Autodesk Inventor part; units mm, degrees
(part 3 of 3)
sketch "Boceto45" plane through (0, 0, 2) normal (0, 0, 1) x (1, 0, 0)
  line L0 (-14.5048, -25.2952) -> (14.5048, -25.2952) construction
  line L1 (14.5048, -25.2952) -> (14.5048, -27.5438) construction
  line L2 (14.5048, -27.5438) -> (-14.5048, -27.5438) construction
  line L3 (-14.5048, -27.5438) -> (-14.5048, -25.2952) construction
  line L4 (-34, -35) -> (34, -35) projected
  spline S0 degree 2 poles (-12.9457, -26.7231) (-12.9457, -26.8722) (-13.0591, -27.1007) (-13.1531, -27.1753) knots 0 0 0 1 2 2 2
  spline S1 degree 2 poles (-13.1531, -27.1753) (-13.2666, -27.2628) (-13.5243, -27.3374) (-13.7285, -27.3374) knots 0 0 0 1 2 2 2
  line L5 (-13.7285, -27.3374) -> (-14.3022, -27.3374)
  line L6 (-14.3022, -27.3374) -> (-14.3022, -25.3374)
  line L7 (-14.3022, -25.3374) -> (-13.7722, -25.3374)
  spline S2 degree 2 poles (-13.7722, -25.3374) (-13.5583, -25.3374) (-13.3444, -25.3649) (-13.2471, -25.4184) knots 0 0 0 1 2 2 2
  spline S3 degree 2 poles (-13.2471, -25.4184) (-13.1385, -25.4751) (-13.0397, -25.6615) (-13.0397, -25.7879) knots 0 0 0 1 2 2 2
  spline S4 degree 2 poles (-13.0397, -25.7879) (-13.0397, -25.9289) (-13.1888, -26.1526) (-13.32, -26.2158) knots 0 0 0 1 2 2 2
  line L8 (-13.32, -26.2158) -> (-13.32, -26.2255)
  spline S5 degree 2 poles (-13.32, -26.2255) (-13.1418, -26.2741) (-12.9457, -26.5318) (-12.9457, -26.7231) knots 0 0 0 1 2 2 2
  spline S6 degree 2 poles (-13.2228, -26.7344) (-13.2228, -26.621) (-13.2876, -26.4751) (-13.3849, -26.4233) knots 0 0 0 1 2 2 2
  spline S7 degree 2 poles (-13.3849, -26.4233) (-13.4481, -26.3908) (-13.5972, -26.3714) (-13.735, -26.3714) knots 0 0 0 1 2 2 2
  line L9 (-13.735, -26.3714) -> (-14.0364, -26.3714)
  line L10 (-14.0364, -26.3714) -> (-14.0364, -27.1104)
  line L11 (-14.0364, -27.1104) -> (-13.8209, -27.1104)
  spline S8 degree 2 poles (-13.8209, -27.1104) (-13.6458, -27.1104) (-13.4448, -27.078) (-13.367, -27.0262) knots 0 0 0 1 2 2 2
  spline S9 degree 2 poles (-13.367, -27.0262) (-13.2925, -26.9727) (-13.2228, -26.8398) (-13.2228, -26.7344) knots 0 0 0 1 2 2 2
  spline S10 degree 2 poles (-13.3168, -25.8252) (-13.3168, -25.7539) (-13.3654, -25.6469) (-13.4189, -25.6161) knots 0 0 0 1 2 2 2
  spline S11 degree 2 poles (-13.4189, -25.6161) (-13.4837, -25.5805) (-13.6409, -25.5643) (-13.782, -25.5643) knots 0 0 0 1 2 2 2
  line L12 (-13.782, -25.5643) -> (-14.0364, -25.5643)
  line L13 (-14.0364, -25.5643) -> (-14.0364, -26.1493)
  line L14 (-14.0364, -26.1493) -> (-13.735, -26.1493)
  spline S12 degree 2 poles (-13.735, -26.1493) (-13.6102, -26.1493) (-13.4918, -26.1234) (-13.4286, -26.0829) knots 0 0 0 1 2 2 2
  spline S13 degree 2 poles (-13.4286, -26.0829) (-13.367, -26.044) (-13.3168, -25.9192) (-13.3168, -25.8252) knots 0 0 0 1 2 2 2
  spline S14 degree 2 poles (-11.9829, -27.3795) (-12.1596, -27.3795) (-12.4221, -27.2871) (-12.5145, -27.1947) knots 0 0 0 1 2 2 2
  spline S15 degree 2 poles (-12.5145, -27.1947) (-12.6199, -27.091) (-12.7058, -26.7993) (-12.7058, -26.5853) knots 0 0 0 1 2 2 2
  line L15 (-12.7058, -26.5853) -> (-12.7058, -25.3374)
  line L16 (-12.7058, -25.3374) -> (-12.44, -25.3374)
  line L17 (-12.44, -25.3374) -> (-12.44, -26.5853)
  spline S16 degree 2 poles (-12.44, -26.5853) (-12.44, -26.7247) (-12.4043, -26.9127) (-12.3541, -26.9889) knots 0 0 0 1 2 2 2
  spline S17 degree 2 poles (-12.3541, -26.9889) (-12.3006, -27.0699) (-12.1158, -27.1526) (-11.9829, -27.1526) knots 0 0 0 1 2 2 2
  spline S18 degree 2 poles (-11.9829, -27.1526) (-11.8581, -27.1526) (-11.6636, -27.0699) (-11.6102, -26.9889) knots 0 0 0 1 2 2 2
  spline S19 degree 2 poles (-11.6102, -26.9889) (-11.5599, -26.9127) (-11.5243, -26.7263) (-11.5243, -26.5918) knots 0 0 0 1 2 2 2
  line L18 (-11.5243, -26.5918) -> (-11.5243, -25.3374)
  line L19 (-11.5243, -25.3374) -> (-11.2585, -25.3374)
  line L20 (-11.2585, -25.3374) -> (-11.2585, -26.5853)
  spline S20 degree 2 poles (-11.2585, -26.5853) (-11.2585, -26.7944) (-11.3427, -27.0926) (-11.4497, -27.1947) knots 0 0 0 1 2 2 2
  spline S21 degree 2 poles (-11.4497, -27.1947) (-11.5453, -27.2887) (-11.7982, -27.3795) (-11.9829, -27.3795) knots 0 0 0 1 2 2 2
  line L21 (-9.3298, -27.3374) -> (-9.675, -27.3374)
  line L22 (-9.675, -27.3374) -> (-10.3071, -26.5416)
  line L23 (-10.3071, -26.5416) -> (-10.6118, -26.5416)
  line L24 (-10.6118, -26.5416) -> (-10.6118, -27.3374)
  line L25 (-10.6118, -27.3374) -> (-10.8776, -27.3374)
  line L26 (-10.8776, -27.3374) -> (-10.8776, -25.3374)
  line L27 (-10.8776, -25.3374) -> (-10.3622, -25.3374)
  spline S22 degree 2 poles (-10.3622, -25.3374) (-10.1904, -25.3374) (-9.9586, -25.3746) (-9.8533, -25.4427) knots 0 0 0 1 2 2 2
  spline S23 degree 2 poles (-9.8533, -25.4427) (-9.7479, -25.5108) (-9.6264, -25.7231) (-9.6264, -25.8803) knots 0 0 0 1 2 2 2
  spline S24 degree 2 poles (-9.6264, -25.8803) (-9.6264, -26.0991) (-9.85, -26.3957) (-10.0413, -26.467) knots 0 0 0 1 2 2 2
  line L28 (-10.0413, -26.467) -> (-9.3298, -27.3374)
  spline S25 degree 2 poles (-9.9035, -25.9014) (-9.9035, -25.8139) (-9.9651, -25.6793) (-10.0299, -25.6356) knots 0 0 0 1 2 2 2
  spline S26 degree 2 poles (-10.0299, -25.6356) (-10.0867, -25.5983) (-10.2374, -25.5675) (-10.3476, -25.5675) knots 0 0 0 1 2 2 2
  line L29 (-10.3476, -25.5675) -> (-10.6118, -25.5675)
  line L30 (-10.6118, -25.5675) -> (-10.6118, -26.3195)
  line L31 (-10.6118, -26.3195) -> (-10.3784, -26.3195)
  spline S27 degree 2 poles (-10.3784, -26.3195) (-10.2633, -26.3195) (-10.0802, -26.279) (-10.017, -26.2158) knots 0 0 0 1 2 2 2
  spline S28 degree 2 poles (-10.017, -26.2158) (-9.9586, -26.1607) (-9.9035, -26.0051) (-9.9035, -25.9014) knots 0 0 0 1 2 2 2
  line L32 (-7.7398, -27.3374) -> (-8.038, -27.3374)
  line L33 (-8.038, -27.3374) -> (-8.923, -25.6129)
  line L34 (-8.923, -25.6129) -> (-8.923, -27.3374)
  line L35 (-8.923, -27.3374) -> (-9.1709, -27.3374)
  line L36 (-9.1709, -27.3374) -> (-9.1709, -25.3374)
  line L37 (-9.1709, -25.3374) -> (-8.7933, -25.3374)
  line L38 (-8.7933, -25.3374) -> (-7.9878, -26.9208)
  line L39 (-7.9878, -26.9208) -> (-7.9878, -25.3374)
  line L40 (-7.9878, -25.3374) -> (-7.7398, -25.3374)
  line L41 (-7.7398, -25.3374) -> (-7.7398, -27.3374)
  line L42 (-6.6588, -26.5837) -> (-7.4157, -26.5837)
  line L43 (-7.4157, -26.5837) -> (-7.4157, -26.3406)
  line L44 (-7.4157, -26.3406) -> (-6.6588, -26.3406)
  line L45 (-6.6588, -26.3406) -> (-6.6588, -26.5837)
  line L46 (-5.6393, -27.3374) -> (-6.414, -27.3374)
  line L47 (-6.414, -27.3374) -> (-6.414, -27.1331)
  line L48 (-6.414, -27.1331) -> (-6.1596, -27.1331)
  line L49 (-6.1596, -27.1331) -> (-6.1596, -25.5416)
  line L50 (-6.1596, -25.5416) -> (-6.414, -25.5416)
  line L51 (-6.414, -25.5416) -> (-6.414, -25.3374)
  line L52 (-6.414, -25.3374) -> (-5.6393, -25.3374)
  line L53 (-5.6393, -25.3374) -> (-5.6393, -25.5416)
  line L54 (-5.6393, -25.5416) -> (-5.8938, -25.5416)
  line L55 (-5.8938, -25.5416) -> (-5.8938, -27.1331)
  line L56 (-5.8938, -27.1331) -> (-5.6393, -27.1331)
  line L57 (-5.6393, -27.1331) -> (-5.6393, -27.3374)
  line L58 (-3.8792, -27.3374) -> (-4.1774, -27.3374)
  line L59 (-4.1774, -27.3374) -> (-5.0623, -25.6129)
  line L60 (-5.0623, -25.6129) -> (-5.0623, -27.3374)
  line L61 (-5.0623, -27.3374) -> (-5.3103, -27.3374)
  line L62 (-5.3103, -27.3374) -> (-5.3103, -25.3374)
  line L63 (-5.3103, -25.3374) -> (-4.9327, -25.3374)
  line L64 (-4.9327, -25.3374) -> (-4.1272, -26.9208)
  line L65 (-4.1272, -26.9208) -> (-4.1272, -25.3374)
  line L66 (-4.1272, -25.3374) -> (-3.8792, -25.3374)
  line L67 (-3.8792, -25.3374) -> (-3.8792, -27.3374)
  line L68 (-2.1482, -27.3374) -> (-2.1482, -25.574)
  line L69 (-2.1482, -25.574) -> (-2.8192, -25.574)
  line L70 (-2.8192, -25.574) -> (-2.8192, -25.3374)
  line L71 (-2.8192, -25.3374) -> (-1.2115, -25.3374)
  line L72 (-1.2115, -25.3374) -> (-1.2115, -25.574)
  line L73 (-1.2115, -25.574) -> (-1.8824, -25.574)
  line L74 (-1.8824, -25.574) -> (-1.8824, -27.3374)
  line L75 (-1.8824, -27.3374) -> (-2.1482, -27.3374)
  line L76 (-1.0089, -27.3374) -> (-1.0089, -25.3374)
  line L77 (-1.0089, -25.3374) -> (0.2424, -25.3374)
  line L78 (0.2424, -25.3374) -> (0.2424, -25.574)
  line L79 (0.2424, -25.574) -> (-0.7431, -25.574)
  line L80 (-0.7431, -25.574) -> (-0.7431, -26.1218)
  line L81 (-0.7431, -26.1218) -> (0.1759, -26.1218)
  line L82 (0.1759, -26.1218) -> (0.1759, -26.3584)
  line L83 (0.1759, -26.3584) -> (-0.7431, -26.3584)
  line L84 (-0.7431, -26.3584) -> (-0.7431, -27.1007)
  line L85 (-0.7431, -27.1007) -> (0.2424, -27.1007)
  line L86 (0.2424, -27.1007) -> (0.2424, -27.3374)
  line L87 (0.2424, -27.3374) -> (-1.0089, -27.3374)
  spline S29 degree 2 poles (1.0916, -27.373) (0.8744, -27.373) (0.5697, -27.2822) (0.4352, -27.2174) knots 0 0 0 1 2 2 2
  line L88 (0.4352, -27.2174) -> (0.4352, -26.8835)
  line L89 (0.4352, -26.8835) -> (0.4547, -26.8835)
  spline S30 degree 2 poles (0.4547, -26.8835) (0.586, -27.0067) (0.9182, -27.1429) (1.0722, -27.1429) knots 0 0 0 1 2 2 2
  spline S31 degree 2 poles (1.0722, -27.1429) (1.2926, -27.1429) (1.5179, -26.9597) (1.5179, -26.809) knots 0 0 0 1 2 2 2
  spline S32 degree 2 poles (1.5179, -26.809) (1.5179, -26.6891) (1.3996, -26.5399) (1.2715, -26.5027) knots 0 0 0 1 2 2 2
  spline S33 degree 2 poles (1.2715, -26.5027) (1.1791, -26.4767) (1.0252, -26.4411) (0.9101, -26.4119) knots 0 0 0 1 2 2 2
  spline S34 degree 2 poles (0.9101, -26.4119) (0.8064, -26.3844) (0.6427, -26.3017) (0.5795, -26.2352) knots 0 0 0 1 2 2 2
  spline S35 degree 2 poles (0.5795, -26.2352) (0.5179, -26.1688) (0.4498, -25.9905) (0.4498, -25.8738) knots 0 0 0 1 2 2 2
  spline S36 degree 2 poles (0.4498, -25.8738) (0.4498, -25.6307) (0.8291, -25.3017) (1.1224, -25.3017) knots 0 0 0 1 2 2 2
  spline S37 degree 2 poles (1.1224, -25.3017) (1.291, -25.3017) (1.5892, -25.3681) (1.7172, -25.4314) knots 0 0 0 1 2 2 2
  line L90 (1.7172, -25.4314) -> (1.7172, -25.749)
  line L91 (1.7172, -25.749) -> (1.6978, -25.749)
  spline S38 degree 2 poles (1.6978, -25.749) (1.6022, -25.6615) (1.3039, -25.5318) (1.1402, -25.5318) knots 0 0 0 1 2 2 2
  spline S39 degree 2 poles (1.1402, -25.5318) (0.9555, -25.5318) (0.727, -25.7053) (0.727, -25.8463) knots 0 0 0 1 2 2 2
  spline S40 degree 2 poles (0.727, -25.8463) (0.727, -25.9727) (0.8615, -26.1234) (0.9879, -26.1575) knots 0 0 0 1 2 2 2
  spline S41 degree 2 poles (0.9879, -26.1575) (1.0722, -26.1801) (1.3169, -26.2385) (1.3979, -26.2628) knots 0 0 0 1 2 2 2
  spline S42 degree 2 poles (1.3979, -26.2628) (1.6038, -26.326) (1.795, -26.5805) (1.795, -26.7669) knots 0 0 0 1 2 2 2
  spline S43 degree 2 poles (1.795, -26.7669) (1.795, -26.8852) (1.6994, -27.1121) (1.6135, -27.1915) knots 0 0 0 1 2 2 2
  spline S44 degree 2 poles (1.6135, -27.1915) (1.5179, -27.279) (1.2748, -27.373) (1.0916, -27.373) knots 0 0 0 1 2 2 2
  line L92 (2.5325, -27.3374) -> (2.5325, -25.574)
  line L93 (2.5325, -25.574) -> (1.8615, -25.574)
  line L94 (1.8615, -25.574) -> (1.8615, -25.3374)
  line L95 (1.8615, -25.3374) -> (3.4693, -25.3374)
  line L96 (3.4693, -25.3374) -> (3.4693, -25.574)
  line L97 (3.4693, -25.574) -> (2.7983, -25.574)
  line L98 (2.7983, -25.574) -> (2.7983, -27.3374)
  line L99 (2.7983, -27.3374) -> (2.5325, -27.3374)
  line L100 (6.2456, -27.3374) -> (5.9798, -27.3374)
  line L101 (5.9798, -27.3374) -> (5.9798, -25.6145)
  line L102 (5.9798, -25.6145) -> (5.4579, -26.7863)
  line L103 (5.4579, -26.7863) -> (5.2958, -26.7863)
  line L104 (5.2958, -26.7863) -> (4.7788, -25.6145)
  line L105 (4.7788, -25.6145) -> (4.7788, -27.3374)
  line L106 (4.7788, -27.3374) -> (4.5308, -27.3374)
  line L107 (4.5308, -27.3374) -> (4.5308, -25.3374)
  line L108 (4.5308, -25.3374) -> (4.8939, -25.3374)
  line L109 (4.8939, -25.3374) -> (5.3931, -26.4508)
  line L110 (5.3931, -26.4508) -> (5.8761, -25.3374)
  line L111 (5.8761, -25.3374) -> (6.2456, -25.3374)
  line L112 (6.2456, -25.3374) -> (6.2456, -27.3374)
  spline S45 degree 2 poles (8.0657, -25.5659) (8.1791, -25.6988) (8.3056, -26.0878) (8.3056, -26.3374) knots 0 0 0 1 2 2 2
  spline S46 degree 2 poles (8.3056, -26.3374) (8.3056, -26.5805) (8.1824, -26.9743) (8.0657, -27.1072) knots 0 0 0 1 2 2 2
  spline S47 degree 2 poles (8.0657, -27.1072) (7.9425, -27.2466) (7.6167, -27.3795) (7.4206, -27.3795) knots 0 0 0 1 2 2 2
  spline S48 degree 2 poles (7.4206, -27.3795) (7.218, -27.3795) (6.8939, -27.2417) (6.7756, -27.1072) knots 0 0 0 1 2 2 2
  spline S49 degree 2 poles (6.7756, -27.1072) (6.6605, -26.9743) (6.5373, -26.5837) (6.5373, -26.3374) knots 0 0 0 1 2 2 2
  spline S50 degree 2 poles (6.5373, -26.3374) (6.5373, -26.0861) (6.6621, -25.7036) (6.7772, -25.5659) knots 0 0 0 1 2 2 2
  spline S51 degree 2 poles (6.7772, -25.5659) (6.8939, -25.433) (7.2197, -25.2952) (7.4206, -25.2952) knots 0 0 0 1 2 2 2
  spline S52 degree 2 poles (7.4206, -25.2952) (7.6249, -25.2952) (7.9522, -25.4378) (8.0657, -25.5659) knots 0 0 0 1 2 2 2
  spline S53 degree 2 poles (8.0284, -26.3374) (8.0284, -26.1396) (7.9425, -25.8333) (7.8647, -25.7328) knots 0 0 0 1 2 2 2
  spline S54 degree 2 poles (7.8647, -25.7328) (7.7853, -25.6291) (7.5616, -25.5254) (7.4223, -25.5254) knots 0 0 0 1 2 2 2
  spline S55 degree 2 poles (7.4223, -25.5254) (7.278, -25.5254) (7.0608, -25.6258) (6.9782, -25.7328) knots 0 0 0 1 2 2 2
  spline S56 degree 2 poles (6.9782, -25.7328) (6.8988, -25.8349) (6.8145, -26.1429) (6.8145, -26.3374) knots 0 0 0 1 2 2 2
  spline S57 degree 2 poles (6.8145, -26.3374) (6.8145, -26.7312) (7.1451, -27.1493) (7.4223, -27.1493) knots 0 0 0 1 2 2 2
  spline S58 degree 2 poles (7.4223, -27.1493) (7.6994, -27.1493) (8.0284, -26.7312) (8.0284, -26.3374) knots 0 0 0 1 2 2 2
  spline S59 degree 2 poles (10.1743, -26.339) (10.1743, -26.6129) (9.9522, -27.0537) (9.7659, -27.1769) knots 0 0 0 1 2 2 2
  spline S60 degree 2 poles (9.7659, -27.1769) (9.6135, -27.2725) (9.3007, -27.3374) (9.0576, -27.3374) knots 0 0 0 1 2 2 2
  line L113 (9.0576, -27.3374) -> (8.5973, -27.3374)
  line L114 (8.5973, -27.3374) -> (8.5973, -25.3374)
  line L115 (8.5973, -25.3374) -> (9.0527, -25.3374)
  spline S61 degree 2 poles (9.0527, -25.3374) (9.3347, -25.3374) (9.6556, -25.4216) (9.7691, -25.4962) knots 0 0 0 1 2 2 2
  spline S62 degree 2 poles (9.7691, -25.4962) (9.962, -25.6242) (10.1743, -26.0472) (10.1743, -26.339) knots 0 0 0 1 2 2 2
  spline S63 degree 2 poles (9.8971, -26.3357) (9.8971, -26.1056) (9.7448, -25.7798) (9.5941, -25.6874) knots 0 0 0 1 2 2 2
  spline S64 degree 2 poles (9.5941, -25.6874) (9.4871, -25.6242) (9.2456, -25.5675) (9.0657, -25.5675) knots 0 0 0 1 2 2 2
  line L116 (9.0657, -25.5675) -> (8.8631, -25.5675)
  line L117 (8.8631, -25.5675) -> (8.8631, -27.1072)
  line L118 (8.8631, -27.1072) -> (9.0657, -27.1072)
  spline S65 degree 2 poles (9.0657, -27.1072) (9.2424, -27.1072) (9.5098, -27.0505) (9.6184, -26.9743) knots 0 0 0 1 2 2 2
  spline S66 degree 2 poles (9.6184, -26.9743) (9.7578, -26.8803) (9.8971, -26.5691) (9.8971, -26.3357) knots 0 0 0 1 2 2 2
  spline S67 degree 2 poles (11.1613, -27.3795) (10.9847, -27.3795) (10.7221, -27.2871) (10.6297, -27.1947) knots 0 0 0 1 2 2 2
  spline S68 degree 2 poles (10.6297, -27.1947) (10.5244, -27.091) (10.4385, -26.7993) (10.4385, -26.5853) knots 0 0 0 1 2 2 2
  line L119 (10.4385, -26.5853) -> (10.4385, -25.3374)
  line L120 (10.4385, -25.3374) -> (10.7043, -25.3374)
  line L121 (10.7043, -25.3374) -> (10.7043, -26.5853)
  spline S69 degree 2 poles (10.7043, -26.5853) (10.7043, -26.7247) (10.7399, -26.9127) (10.7902, -26.9889) knots 0 0 0 1 2 2 2
  spline S70 degree 2 poles (10.7902, -26.9889) (10.8437, -27.0699) (11.0284, -27.1526) (11.1613, -27.1526) knots 0 0 0 1 2 2 2
  spline S71 degree 2 poles (11.1613, -27.1526) (11.2861, -27.1526) (11.4806, -27.0699) (11.5341, -26.9889) knots 0 0 0 1 2 2 2
  spline S72 degree 2 poles (11.5341, -26.9889) (11.5843, -26.9127) (11.62, -26.7263) (11.62, -26.5918) knots 0 0 0 1 2 2 2
  line L122 (11.62, -26.5918) -> (11.62, -25.3374)
  line L123 (11.62, -25.3374) -> (11.8858, -25.3374)
  line L124 (11.8858, -25.3374) -> (11.8858, -26.5853)
  spline S73 degree 2 poles (11.8858, -26.5853) (11.8858, -26.7944) (11.8015, -27.0926) (11.6945, -27.1947) knots 0 0 0 1 2 2 2
  spline S74 degree 2 poles (11.6945, -27.1947) (11.5989, -27.2887) (11.3461, -27.3795) (11.1613, -27.3795) knots 0 0 0 1 2 2 2
  line L125 (13.4255, -27.3374) -> (12.2667, -27.3374)
  line L126 (12.2667, -27.3374) -> (12.2667, -25.3374)
  line L127 (12.2667, -25.3374) -> (12.5325, -25.3374)
  line L128 (12.5325, -25.3374) -> (12.5325, -27.1007)
  line L129 (12.5325, -27.1007) -> (13.4255, -27.1007)
  line L130 (13.4255, -27.1007) -> (13.4255, -27.3374)
  line L131 (13.6346, -27.3374) -> (13.6346, -25.3374)
  line L132 (13.6346, -25.3374) -> (14.8858, -25.3374)
  line L133 (14.8858, -25.3374) -> (14.8858, -25.574)
  line L134 (14.8858, -25.574) -> (13.9004, -25.574)
  line L135 (13.9004, -25.574) -> (13.9004, -26.1218)
  line L136 (13.9004, -26.1218) -> (14.8193, -26.1218)
  line L137 (14.8193, -26.1218) -> (14.8193, -26.3584)
  line L138 (14.8193, -26.3584) -> (13.9004, -26.3584)
  line L139 (13.9004, -26.3584) -> (13.9004, -27.1007)
  line L140 (13.9004, -27.1007) -> (14.8858, -27.1007)
  line L141 (14.8858, -27.1007) -> (14.8858, -27.3374)
  line L142 (14.8858, -27.3374) -> (13.6346, -27.3374)
  point P0 (0, 0)
  point P1 (0, -25.2952)
  constraints: 1 midpoint, 1 vertical alignment, 2 other
extrude "Extrusión18" add sketch "Boceto45" along normal blind 0.001
